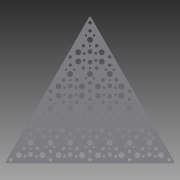
# Autodesk Inventor part: grid16-lightpipe
Saved by Autodesk Inventor 2013 (Build 170138000, 138)
## iProperties
Created: 2013-03-05
Part Number: grid16-lightpipe
Material: Generic
Document SubType Name: Modeling
Designer: Beth Scott
Density: 1 g/cm^3
Author: Beth Scott
Autodesk Inventor part; units mm, degrees
(part 1 of 2)
ref_plane "YZ Plane" through (0, 0, 0) normal (1, 0, 0) x (0, 1, 0)
ref_plane "XZ Plane" through (0, 0, 0) normal (0, 1, 0) x (-1, 0, 0)
ref_plane "XY Plane" through (0, 0, 0) normal (0, 0, 1) x (1, 0, 0)
sketch "Triangle 1mm" plane through (0, 0, 0) normal (0, 0, 1) x (1, 0, 0)
  line L0 (0, 0) -> (16.6665, 28.8672) construction
  line L1 (16.6665, 28.8672) -> (33.333, 0) construction
  line L2 (33.333, 0) -> (0, 0) construction
  line L3 (33.333, 0) -> (8.3332, 14.4336) construction
  line L4 (0, 0) -> (24.9997, 14.4336) construction
  line L5 (16.6665, 28.8672) -> (16.6665, 0) construction
  line L6 (0, 14.4336) -> (33.333, 14.4336) construction
  line L7 (0, 19.4336) -> (33.333, 19.4336) construction
  line L8 (0, 9.4336) -> (33.333, 9.4336) construction
  line L9 (16.6665, 19.4336) -> (16.6665, 14.4336) construction
  line L10 (16.6665, 14.4336) -> (16.6665, 9.4336) construction
  circle A0 centre (16.6665, 14.4336) radius 2.5
  circle A1 centre (16.6665, 14.4336) radius 14.4336 construction
  circle A2 centre (6.7821, 3.9156) radius 2.5
  circle A3 centre (26.5509, 3.9156) radius 2.5
  circle A4 centre (16.6665, 14.4336) radius 10 construction
  circle A5 centre (16.6665, 4.4336) radius 2
  circle A6 centre (16.6665, 14.4336) radius 7.5 construction
  circle A7 centre (11.0763, 9.4336) radius 1.5
  circle A8 centre (22.2567, 9.4336) radius 1.5
  circle A9 centre (16.6665, 9.4336) radius 1
  circle A10 centre (16.6665, 21.9336) radius 1.5
  circle A11 centre (16.6665, 14.4336) radius 5 construction
  line L11 (5.4465, 9.4336) -> (22.2567, 19.4336) construction
  line L12 (27.8865, 9.4336) -> (11.0763, 19.4336) construction
  circle A12 centre (20.046, 18.1186) radius 1
  circle A13 centre (13.287, 18.1186) radius 1
  circle A14 centre (16.6665, 14.4336) radius 12.5 construction
  circle A15 centre (21.5432, 2.9241) radius 1.25
  circle A16 centre (11.7898, 2.9241) radius 1.25
  line L13 (16.6665, 4.4336) -> (21.5432, 2.9241) construction
  line L14 (21.5432, 2.9241) -> (26.5509, 3.9156) construction
  line L15 (6.7821, 3.9156) -> (11.7898, 2.9241) construction
  line L16 (11.7898, 2.9241) -> (16.6665, 4.4336) construction
  circle A17 centre (0, 0) radius 2.75 construction
  circle A18 centre (33.333, 0) radius 2.75 construction
  circle A19 centre (16.6665, 28.8672) radius 2.75 construction
  point P0 (16.9666, 9.7956)
  dimension "d55" = 20
  dimension "d14" = 33.333
  dimension "d31" = 10
  dimension "d43" = 5
  dimension "d54" = 5
  dimension "d56" = 4
  dimension "d57" = 15
  dimension "d58" = 3
  dimension "d59" = 2
  dimension "d60" = 25
  dimension "d61" = 2.5
  dimension "d64" = 5.5
  measures "d14" distance of L1.end L0.start
  measures "d31" distance of L8.start L7.start
  measures "d43" diameter of A0
  measures "d54" diameter of A2
  measures "d56" diameter of A5
  measures "d57" diameter of A6
  measures "d58" diameter of A7
  measures "d59" diameter of A9
  measures "d60" diameter of A14
  measures "d61" diameter of A15
  measures "d64" diameter of A17
sketch "Tri16 1mm" plane through (0, 0, 0) normal (0, 0, 1) x (1, 0, 0)
  line L0 (0, 0) -> (16.6665, 28.8672) construction
  line L1 (16.6665, 28.8672) -> (33.333, 0) construction
  line L2 (33.333, 0) -> (0, 0) construction
  line L3 (33.333, 0) -> (8.3333, 14.4336) construction
  line L4 (0, 0) -> (24.9998, 14.4336) construction
  line L5 (16.6665, 28.8672) -> (16.6665, 0) construction
  line L6 (0, 14.4336) -> (33.333, 14.4336) construction
  line L7 (0, 19.4336) -> (33.333, 19.4336) construction
  line L8 (0, 9.4336) -> (33.333, 9.4336) construction
  line L9 (16.6665, 19.4336) -> (16.6665, 14.4336) construction
  line L10 (16.6665, 14.4336) -> (16.6665, 9.4336) construction
  circle A0 centre (16.6665, 14.4336) radius 2.5
  circle A1 centre (16.6665, 14.4336) radius 14.4336 construction
  circle A2 centre (6.7821, 3.9156) radius 2.5
  circle A3 centre (26.5509, 3.9156) radius 2.5
  circle A4 centre (16.6665, 14.4336) radius 10 construction
  circle A5 centre (16.6665, 4.4336) radius 2
  circle A6 centre (16.6665, 14.4336) radius 7.5 construction
  circle A7 centre (11.0763, 9.4336) radius 1.5
  circle A8 centre (22.2567, 9.4336) radius 1.5
  circle A9 centre (16.6665, 9.4336) radius 1
  circle A10 centre (16.6665, 21.9336) radius 1.5
  circle A11 centre (16.6665, 14.4336) radius 5 construction
  line L11 (5.4465, 9.4336) -> (22.2567, 19.4336) construction
  line L12 (27.8865, 9.4336) -> (11.0763, 19.4336) construction
  circle A12 centre (20.046, 18.1186) radius 1
  circle A13 centre (13.287, 18.1186) radius 1
  circle A14 centre (16.6665, 14.4336) radius 12.5 construction
  circle A15 centre (21.5432, 2.9241) radius 1.25
  circle A16 centre (11.7898, 2.9241) radius 1.25
  line L13 (16.6665, 4.4336) -> (21.5432, 2.9241) construction
  line L14 (21.5432, 2.9241) -> (26.5509, 3.9156) construction
  line L15 (6.7821, 3.9156) -> (11.7898, 2.9241) construction
  line L16 (11.7898, 2.9241) -> (16.6665, 4.4336) construction
  circle A17 centre (0, 0) radius 2.75 construction
  circle A18 centre (33.333, 0) radius 2.75 construction
  circle A19 centre (16.6665, 28.8672) radius 2.75 construction
  line L17 (33.333, 0) -> (49.9995, 28.8672) construction
  line L18 (49.9995, 28.8672) -> (66.666, 0) construction
  line L19 (66.666, 0) -> (33.333, 0) construction
  line L20 (66.666, 0) -> (41.6663, 14.4336) construction
  line L21 (33.333, 0) -> (58.3328, 14.4336) construction
  line L22 (49.9995, 28.8672) -> (49.9995, 0) construction
  line L23 (33.333, 14.4336) -> (66.666, 14.4336) construction
  line L24 (33.333, 19.4336) -> (66.666, 19.4336) construction
  line L25 (33.333, 9.4336) -> (66.666, 9.4336) construction
  line L26 (49.9995, 19.4336) -> (49.9995, 14.4336) construction
  line L27 (49.9995, 14.4336) -> (49.9995, 9.4336) construction
  circle A20 centre (49.9995, 14.4336) radius 2.5
  circle A21 centre (49.9995, 14.4336) radius 14.4336 construction
  circle A22 centre (40.1151, 3.9156) radius 2.5
  circle A23 centre (59.8839, 3.9156) radius 2.5
  circle A24 centre (49.9995, 14.4336) radius 10 construction
  circle A25 centre (49.9995, 4.4336) radius 2
  circle A26 centre (49.9995, 14.4336) radius 7.5 construction
  circle A27 centre (44.4093, 9.4336) radius 1.5
  circle A28 centre (55.5897, 9.4336) radius 1.5
  circle A29 centre (49.9995, 9.4336) radius 1
  circle A30 centre (49.9995, 21.9336) radius 1.5
  circle A31 centre (49.9995, 14.4336) radius 5 construction
  line L28 (38.7795, 9.4336) -> (55.5897, 19.4336) construction
  line L29 (61.2195, 9.4336) -> (44.4093, 19.4336) construction
  circle A32 centre (53.379, 18.1186) radius 1
  circle A33 centre (46.62, 18.1186) radius 1
  circle A34 centre (49.9995, 14.4336) radius 12.5 construction
  circle A35 centre (54.8762, 2.9241) radius 1.25
  circle A36 centre (45.1228, 2.9241) radius 1.25
  line L30 (49.9995, 4.4336) -> (54.8762, 2.9241) construction
  line L31 (54.8762, 2.9241) -> (59.8839, 3.9156) construction
  line L32 (40.1151, 3.9156) -> (45.1228, 2.9241) construction
  line L33 (45.1228, 2.9241) -> (49.9995, 4.4336) construction
  circle A37 centre (33.333, 0) radius 2.75 construction
  circle A38 centre (66.666, 0) radius 2.75 construction
  circle A39 centre (49.9995, 28.8672) radius 2.75 construction
  line L34 (49.9995, 28.8672) -> (33.333, 0) construction
  line L35 (33.333, 0) -> (16.6665, 28.8672) construction
  line L36 (16.6665, 28.8672) -> (49.9995, 28.8672) construction
  line L37 (16.6665, 28.8672) -> (41.6663, 14.4336) construction
  line L38 (49.9995, 28.8672) -> (24.9998, 14.4336) construction
  line L39 (33.333, 0) -> (33.333, 28.8672) construction
  line L40 (49.9995, 14.4336) -> (16.6665, 14.4336) construction
  line L41 (49.9995, 9.4336) -> (16.6665, 9.4336) construction
  line L42 (49.9995, 19.4336) -> (16.6665, 19.4336) construction
  line L43 (33.333, 9.4336) -> (33.333, 14.4336) construction
  line L44 (33.333, 14.4336) -> (33.333, 19.4336) construction
  circle A40 centre (33.333, 14.4336) radius 2.5
  circle A41 centre (33.333, 14.4336) radius 14.4336 construction
  circle A42 centre (43.2174, 24.9516) radius 2.5
  circle A43 centre (23.4486, 24.9516) radius 2.5
  circle A44 centre (33.333, 14.4336) radius 10 construction
  circle A45 centre (33.333, 24.4336) radius 2
  circle A46 centre (33.333, 14.4336) radius 7.5 construction
  circle A47 centre (38.9232, 19.4336) radius 1.5
  circle A48 centre (27.7428, 19.4336) radius 1.5
  circle A49 centre (33.333, 19.4336) radius 1
  circle A50 centre (33.333, 6.9336) radius 1.5
  circle A51 centre (33.333, 14.4336) radius 5 construction
  line L45 (44.553, 19.4336) -> (27.7428, 9.4336) construction
  line L46 (22.113, 19.4336) -> (38.9232, 9.4336) construction
  circle A52 centre (29.9535, 10.7487) radius 1
  circle A53 centre (36.7125, 10.7487) radius 1
  circle A54 centre (33.333, 14.4336) radius 12.5 construction
  circle A55 centre (28.4563, 25.9431) radius 1.25
  circle A56 centre (38.2097, 25.9431) radius 1.25
  line L47 (33.333, 24.4336) -> (28.4563, 25.9431) construction
  line L48 (28.4563, 25.9431) -> (23.4486, 24.9516) construction
  line L49 (43.2174, 24.9516) -> (38.2097, 25.9431) construction
  line L50 (38.2097, 25.9431) -> (33.333, 24.4336) construction
  circle A57 centre (49.9995, 28.8672) radius 2.75 construction
  circle A58 centre (16.6665, 28.8672) radius 2.75 construction
  circle A59 centre (33.333, 0) radius 2.75 construction
  line L51 (83.3325, 28.8672) -> (66.666, 0) construction
  line L52 (66.666, 0) -> (49.9995, 28.8672) construction
  line L53 (49.9995, 28.8672) -> (83.3325, 28.8672) construction
  line L54 (49.9995, 28.8672) -> (74.9993, 14.4336) construction
  line L55 (83.3325, 28.8672) -> (58.3328, 14.4336) construction
  line L56 (66.666, 0) -> (66.666, 28.8672) construction
  line L57 (83.3325, 14.4336) -> (49.9995, 14.4336) construction
  line L58 (83.3325, 9.4336) -> (49.9995, 9.4336) construction
  line L59 (83.3325, 19.4336) -> (49.9995, 19.4336) construction
  line L60 (66.666, 9.4336) -> (66.666, 14.4336) construction
  line L61 (66.666, 14.4336) -> (66.666, 19.4336) construction
  circle A60 centre (66.666, 14.4336) radius 2.5
  circle A61 centre (66.666, 14.4336) radius 14.4336 construction
  circle A62 centre (76.5504, 24.9516) radius 2.5
  circle A63 centre (56.7816, 24.9516) radius 2.5
  circle A64 centre (66.666, 14.4336) radius 10 construction
  circle A65 centre (66.666, 24.4336) radius 2
  circle A66 centre (66.666, 14.4336) radius 7.5 construction
  circle A67 centre (72.2562, 19.4336) radius 1.5
  circle A68 centre (61.0758, 19.4336) radius 1.5
  circle A69 centre (66.666, 19.4336) radius 1
  circle A70 centre (66.666, 6.9336) radius 1.5
  circle A71 centre (66.666, 14.4336) radius 5 construction
  line L62 (77.886, 19.4336) -> (61.0758, 9.4336) construction
  line L63 (55.446, 19.4336) -> (72.2562, 9.4336) construction
  circle A72 centre (63.2865, 10.7487) radius 1
  circle A73 centre (70.0455, 10.7487) radius 1
  circle A74 centre (66.666, 14.4336) radius 12.5 construction
  circle A75 centre (61.7893, 25.9431) radius 1.25
  circle A76 centre (71.5427, 25.9431) radius 1.25
  line L64 (66.666, 24.4336) -> (61.7893, 25.9431) construction
  line L65 (61.7893, 25.9431) -> (56.7816, 24.9516) construction
  line L66 (76.5504, 24.9516) -> (71.5427, 25.9431) construction
  line L67 (71.5427, 25.9431) -> (66.666, 24.4336) construction
  circle A77 centre (83.3325, 28.8672) radius 2.75 construction
  circle A78 centre (49.9995, 28.8672) radius 2.75 construction
  circle A79 centre (66.666, 0) radius 2.75 construction
  line L68 (66.666, 0) -> (83.3325, 28.8672) construction
  line L69 (83.3325, 28.8672) -> (99.999, 0) construction
  line L70 (99.999, 0) -> (66.666, 0) construction
  line L71 (99.999, 0) -> (74.9993, 14.4336) construction
  line L72 (66.666, 0) -> (91.6658, 14.4336) construction
  line L73 (83.3325, 28.8672) -> (83.3325, 0) construction
  line L74 (66.666, 14.4336) -> (99.999, 14.4336) construction
  line L75 (66.666, 19.4336) -> (99.999, 19.4336) construction
  line L76 (66.666, 9.4336) -> (99.999, 9.4336) construction
  line L77 (83.3325, 19.4336) -> (83.3325, 14.4336) construction
  line L78 (83.3325, 14.4336) -> (83.3325, 9.4336) construction
  circle A80 centre (83.3325, 14.4336) radius 2.5
  circle A81 centre (83.3325, 14.4336) radius 14.4336 construction
  circle A82 centre (73.4481, 3.9156) radius 2.5
  circle A83 centre (93.2169, 3.9156) radius 2.5
  circle A84 centre (83.3325, 14.4336) radius 10 construction
  circle A85 centre (83.3325, 4.4336) radius 2
  circle A86 centre (83.3325, 14.4336) radius 7.5 construction
  circle A87 centre (77.7423, 9.4336) radius 1.5
  circle A88 centre (88.9227, 9.4336) radius 1.5
  circle A89 centre (83.3325, 9.4336) radius 1
  circle A90 centre (83.3325, 21.9336) radius 1.5
  circle A91 centre (83.3325, 14.4336) radius 5 construction
  line L79 (72.1125, 9.4336) -> (88.9227, 19.4336) construction
  line L80 (94.5525, 9.4336) -> (77.7423, 19.4336) construction
  circle A92 centre (86.712, 18.1186) radius 1
  circle A93 centre (79.953, 18.1186) radius 1
  circle A94 centre (83.3325, 14.4336) radius 12.5 construction
  circle A95 centre (88.2092, 2.9241) radius 1.25
  circle A96 centre (78.4558, 2.9241) radius 1.25
  line L81 (83.3325, 4.4336) -> (88.2092, 2.9241) construction
  line L82 (88.2092, 2.9241) -> (93.2169, 3.9156) construction
  line L83 (73.4481, 3.9156) -> (78.4558, 2.9241) construction
  line L84 (78.4558, 2.9241) -> (83.3325, 4.4336) construction
  circle A97 centre (66.666, 0) radius 2.75 construction
  circle A98 centre (99.999, 0) radius 2.75 construction
  circle A99 centre (83.3325, 28.8672) radius 2.75 construction
  line L85 (99.999, 0) -> (116.6655, 28.8672) construction
  line L86 (116.6655, 28.8672) -> (133.332, 0) construction
  line L87 (133.332, 0) -> (99.999, 0) construction
  line L88 (133.332, 0) -> (108.3323, 14.4336) construction
  line L89 (99.999, 0) -> (124.9988, 14.4336) construction
  line L90 (116.6655, 28.8672) -> (116.6655, 0) construction
  line L91 (99.999, 14.4336) -> (133.332, 14.4336) construction
  line L92 (99.999, 19.4336) -> (133.332, 19.4336) construction
  line L93 (99.999, 9.4336) -> (133.332, 9.4336) construction
  line L94 (116.6655, 19.4336) -> (116.6655, 14.4336) construction
  line L95 (116.6655, 14.4336) -> (116.6655, 9.4336) construction
  circle A100 centre (116.6655, 14.4336) radius 2.5
  circle A101 centre (116.6655, 14.4336) radius 14.4336 construction
  circle A102 centre (106.7811, 3.9156) radius 2.5
  circle A103 centre (126.5499, 3.9156) radius 2.5
  circle A104 centre (116.6655, 14.4336) radius 10 construction
  circle A105 centre (116.6655, 4.4336) radius 2
  circle A106 centre (116.6655, 14.4336) radius 7.5 construction
  circle A107 centre (111.0753, 9.4336) radius 1.5
  circle A108 centre (122.2557, 9.4336) radius 1.5
  circle A109 centre (116.6655, 9.4336) radius 1
  circle A110 centre (116.6655, 21.9336) radius 1.5
  circle A111 centre (116.6655, 14.4336) radius 5 construction
  line L96 (105.4455, 9.4336) -> (122.2557, 19.4336) construction
  line L97 (127.8855, 9.4336) -> (111.0753, 19.4336) construction
  circle A112 centre (120.045, 18.1186) radius 1
  circle A113 centre (113.286, 18.1186) radius 1
  circle A114 centre (116.6655, 14.4336) radius 12.5 construction
  circle A115 centre (121.5422, 2.9241) radius 1.25
  circle A116 centre (111.7888, 2.9241) radius 1.25
  line L98 (116.6655, 4.4336) -> (121.5422, 2.9241) construction
  line L99 (121.5422, 2.9241) -> (126.5499, 3.9156) construction
  line L100 (106.7811, 3.9156) -> (111.7888, 2.9241) construction
  line L101 (111.7888, 2.9241) -> (116.6655, 4.4336) construction
  circle A117 centre (99.999, 0) radius 2.75 construction
  circle A118 centre (133.332, 0) radius 2.75 construction
  circle A119 centre (116.6655, 28.8672) radius 2.75 construction
  line L102 (116.6655, 28.8672) -> (99.999, 0) construction
  line L103 (99.999, 0) -> (83.3325, 28.8672) construction
  line L104 (83.3325, 28.8672) -> (116.6655, 28.8672) construction
  line L105 (83.3325, 28.8672) -> (108.3323, 14.4336) construction
  line L106 (116.6655, 28.8672) -> (91.6658, 14.4336) construction
  line L107 (99.999, 0) -> (99.999, 28.8672) construction
  line L108 (116.6655, 14.4336) -> (83.3325, 14.4336) construction
  line L109 (116.6655, 9.4336) -> (83.3325, 9.4336) construction
  line L110 (116.6655, 19.4336) -> (83.3325, 19.4336) construction
  line L111 (99.999, 9.4336) -> (99.999, 14.4336) construction
  line L112 (99.999, 14.4336) -> (99.999, 19.4336) construction
  circle A120 centre (99.999, 14.4336) radius 2.5
  circle A121 centre (99.999, 14.4336) radius 14.4336 construction
  circle A122 centre (109.8834, 24.9516) radius 2.5
  circle A123 centre (90.1146, 24.9516) radius 2.5
  circle A124 centre (99.999, 14.4336) radius 10 construction
  circle A125 centre (99.999, 24.4336) radius 2
  circle A126 centre (99.999, 14.4336) radius 7.5 construction
  circle A127 centre (105.5892, 19.4336) radius 1.5
  circle A128 centre (94.4088, 19.4336) radius 1.5
  circle A129 centre (99.999, 19.4336) radius 1
  circle A130 centre (99.999, 6.9336) radius 1.5
  circle A131 centre (99.999, 14.4336) radius 5 construction
  line L113 (111.219, 19.4336) -> (94.4088, 9.4336) construction
  line L114 (88.779, 19.4336) -> (105.5892, 9.4336) construction
  circle A132 centre (96.6195, 10.7487) radius 1
  circle A133 centre (103.3785, 10.7487) radius 1
  circle A134 centre (99.999, 14.4336) radius 12.5 construction
  circle A135 centre (95.1223, 25.9431) radius 1.25
  circle A136 centre (104.8757, 25.9431) radius 1.25
  line L115 (99.999, 24.4336) -> (95.1223, 25.9431) construction
  line L116 (95.1223, 25.9431) -> (90.1146, 24.9516) construction
  line L117 (109.8834, 24.9516) -> (104.8757, 25.9431) construction
  line L118 (104.8757, 25.9431) -> (99.999, 24.4336) construction
  circle A137 centre (116.6655, 28.8672) radius 2.75 construction
  circle A138 centre (83.3325, 28.8672) radius 2.75 construction
  circle A139 centre (99.999, 0) radius 2.75 construction
  line L119 (16.6665, 28.8672) -> (33.333, 57.7344) construction
  line L120 (33.333, 57.7344) -> (49.9995, 28.8672) construction
  line L121 (49.9995, 28.8672) -> (16.6665, 28.8672) construction
  line L122 (49.9995, 28.8672) -> (24.9998, 43.3008) construction
  line L123 (16.6665, 28.8672) -> (41.6663, 43.3008) construction
  line L124 (33.333, 57.7344) -> (33.333, 28.8672) construction
  line L125 (16.6665, 43.3008) -> (49.9995, 43.3008) construction
  line L126 (16.6665, 48.3008) -> (49.9995, 48.3008) construction
  line L127 (16.6665, 38.3008) -> (49.9995, 38.3008) construction
  line L128 (33.333, 48.3008) -> (33.333, 43.3008) construction
  line L129 (33.333, 43.3008) -> (33.333, 38.3008) construction
  circle A140 centre (33.333, 43.3008) radius 2.5
  circle A141 centre (33.333, 43.3008) radius 14.4336 construction
  circle A142 centre (23.4486, 32.7829) radius 2.5
  circle A143 centre (43.2174, 32.7829) radius 2.5
  circle A144 centre (33.333, 43.3008) radius 10 construction
  circle A145 centre (33.333, 33.3008) radius 2
  circle A146 centre (33.333, 43.3008) radius 7.5 construction
  circle A147 centre (27.7428, 38.3008) radius 1.5
  circle A148 centre (38.9232, 38.3008) radius 1.5
  circle A149 centre (33.333, 38.3008) radius 1
  circle A150 centre (33.333, 50.8008) radius 1.5
  circle A151 centre (33.333, 43.3008) radius 5 construction
  line L130 (22.113, 38.3008) -> (38.9232, 48.3008) construction
  line L131 (44.553, 38.3008) -> (27.7428, 48.3008) construction
  circle A152 centre (36.7125, 46.9858) radius 1
  circle A153 centre (29.9535, 46.9858) radius 1
  circle A154 centre (33.333, 43.3008) radius 12.5 construction
  circle A155 centre (38.2097, 31.7914) radius 1.25
  circle A156 centre (28.4563, 31.7914) radius 1.25
  line L132 (33.333, 33.3008) -> (38.2097, 31.7914) construction
  line L133 (38.2097, 31.7914) -> (43.2174, 32.7829) construction
  line L134 (23.4486, 32.7829) -> (28.4563, 31.7914) construction
  line L135 (28.4563, 31.7914) -> (33.333, 33.3008) construction
  circle A157 centre (16.6665, 28.8672) radius 2.75 construction
  circle A158 centre (49.9995, 28.8672) radius 2.75 construction
  circle A159 centre (33.333, 57.7344) radius 2.75 construction
  line L136 (33.333, 57.7344) -> (49.9995, 86.6017) construction
  line L137 (49.9995, 86.6017) -> (66.666, 57.7344) construction
  line L138 (66.666, 57.7344) -> (33.333, 57.7344) construction
  line L139 (66.666, 57.7344) -> (41.6663, 72.1681) construction
  line L140 (33.333, 57.7344) -> (58.3328, 72.1681) construction
  line L141 (49.9995, 86.6017) -> (49.9995, 57.7344) construction
  line L142 (33.333, 72.1681) -> (66.666, 72.1681) construction
  line L143 (33.333, 77.1681) -> (66.666, 77.1681) construction
  line L144 (33.333, 67.1681) -> (66.666, 67.1681) construction
  line L145 (49.9995, 77.1681) -> (49.9995, 72.1681) construction
  line L146 (49.9995, 72.1681) -> (49.9995, 67.1681) construction
  circle A160 centre (49.9995, 72.1681) radius 2.5
  circle A161 centre (49.9995, 72.1681) radius 14.4336 construction
  circle A162 centre (40.1151, 61.6501) radius 2.5
  circle A163 centre (59.8839, 61.6501) radius 2.5
  circle A164 centre (49.9995, 72.1681) radius 10 construction
  circle A165 centre (49.9995, 62.1681) radius 2
  circle A166 centre (49.9995, 72.1681) radius 7.5 construction
  circle A167 centre (44.4093, 67.1681) radius 1.5
  circle A168 centre (55.5897, 67.1681) radius 1.5
  circle A169 centre (49.9995, 67.1681) radius 1
  circle A170 centre (49.9995, 79.6681) radius 1.5
  circle A171 centre (49.9995, 72.1681) radius 5 construction
  line L147 (38.7795, 67.1681) -> (55.5897, 77.1681) construction
  line L148 (61.2195, 67.1681) -> (44.4093, 77.1681) construction
  circle A172 centre (53.379, 75.853) radius 1
  circle A173 centre (46.62, 75.853) radius 1
  circle A174 centre (49.9995, 72.1681) radius 12.5 construction
  circle A175 centre (54.8762, 60.6586) radius 1.25
  circle A176 centre (45.1228, 60.6586) radius 1.25
  line L149 (49.9995, 62.1681) -> (54.8762, 60.6586) construction
  line L150 (54.8762, 60.6586) -> (59.8839, 61.6501) construction
  line L151 (40.1151, 61.6501) -> (45.1228, 60.6586) construction
  line L152 (45.1228, 60.6586) -> (49.9995, 62.1681) construction
  circle A177 centre (33.333, 57.7344) radius 2.75 construction
  circle A178 centre (66.666, 57.7344) radius 2.75 construction
  circle A179 centre (49.9995, 86.6017) radius 2.75 construction
  line L153 (49.9995, 86.6017) -> (66.666, 115.4689) construction
  line L154 (66.666, 115.4689) -> (83.3325, 86.6017) construction
  line L155 (83.3325, 86.6017) -> (49.9995, 86.6017) construction
  line L156 (83.3325, 86.6017) -> (58.3328, 101.0353) construction
  line L157 (49.9995, 86.6017) -> (74.9993, 101.0353) construction
  line L158 (66.666, 115.4689) -> (66.666, 86.6017) construction
  line L159 (49.9995, 101.0353) -> (83.3325, 101.0353) construction
  line L160 (49.9995, 106.0353) -> (83.3325, 106.0353) construction
  line L161 (49.9995, 96.0353) -> (83.3325, 96.0353) construction
  line L162 (66.666, 106.0353) -> (66.666, 101.0353) construction
  line L163 (66.666, 101.0353) -> (66.666, 96.0353) construction
  circle A180 centre (66.666, 101.0353) radius 2.5
  circle A181 centre (66.666, 101.0353) radius 14.4336 construction
  circle A182 centre (56.7816, 90.5173) radius 2.5
  circle A183 centre (76.5504, 90.5173) radius 2.5
  circle A184 centre (66.666, 101.0353) radius 10 construction
  circle A185 centre (66.666, 91.0353) radius 2
  circle A186 centre (66.666, 101.0353) radius 7.5 construction
  circle A187 centre (61.0758, 96.0353) radius 1.5
  circle A188 centre (72.2562, 96.0353) radius 1.5
  circle A189 centre (66.666, 96.0353) radius 1
  circle A190 centre (66.666, 108.5353) radius 1.5
  circle A191 centre (66.666, 101.0353) radius 5 construction
  line L164 (55.446, 96.0353) -> (72.2562, 106.0353) construction
  line L165 (77.886, 96.0353) -> (61.0758, 106.0353) construction
  circle A192 centre (70.0455, 104.7202) radius 1
  circle A193 centre (63.2865, 104.7202) radius 1
  circle A194 centre (66.666, 101.0353) radius 12.5 construction
  circle A195 centre (71.5427, 89.5258) radius 1.25
  circle A196 centre (61.7893, 89.5258) radius 1.25
  line L166 (66.666, 91.0353) -> (71.5427, 89.5258) construction
  line L167 (71.5427, 89.5258) -> (76.5504, 90.5173) construction
  line L168 (56.7816, 90.5173) -> (61.7893, 89.5258) construction
  line L169 (61.7893, 89.5258) -> (66.666, 91.0353) construction
  circle A197 centre (49.9995, 86.6017) radius 2.75 construction
  circle A198 centre (83.3325, 86.6017) radius 2.75 construction
  circle A199 centre (66.666, 115.4689) radius 2.75 construction
  line L170 (66.666, 57.7344) -> (49.9995, 28.8672) construction
  line L171 (49.9995, 28.8672) -> (33.333, 57.7344) construction
  line L172 (33.333, 57.7344) -> (66.666, 57.7344) construction
  line L173 (33.333, 57.7344) -> (58.3328, 43.3008) construction
  line L174 (66.666, 57.7344) -> (41.6663, 43.3008) construction
  line L175 (49.9995, 28.8672) -> (49.9995, 57.7344) construction
  line L176 (66.666, 43.3008) -> (33.333, 43.3008) construction
  line L177 (66.666, 38.3008) -> (33.333, 38.3008) construction
  line L178 (66.666, 48.3008) -> (33.333, 48.3008) construction
  line L179 (49.9995, 38.3008) -> (49.9995, 43.3008) construction
  line L180 (49.9995, 43.3008) -> (49.9995, 48.3008) construction
  circle A200 centre (49.9995, 43.3008) radius 2.5
  circle A201 centre (49.9995, 43.3008) radius 14.4336 construction
  circle A202 centre (59.8839, 53.8188) radius 2.5
  circle A203 centre (40.1151, 53.8188) radius 2.5
  circle A204 centre (49.9995, 43.3008) radius 10 construction
  circle A205 centre (49.9995, 53.3008) radius 2
  circle A206 centre (49.9995, 43.3008) radius 7.5 construction
  circle A207 centre (55.5897, 48.3008) radius 1.5
  circle A208 centre (44.4093, 48.3008) radius 1.5
  circle A209 centre (49.9995, 48.3008) radius 1
  circle A210 centre (49.9995, 35.8008) radius 1.5
  circle A211 centre (49.9995, 43.3008) radius 5 construction
  line L181 (61.2195, 48.3008) -> (44.4093, 38.3008) construction
  line L182 (38.7795, 48.3008) -> (55.5897, 38.3008) construction
  circle A212 centre (46.62, 39.6159) radius 1
  circle A213 centre (53.379, 39.6159) radius 1
  circle A214 centre (49.9995, 43.3008) radius 12.5 construction
  circle A215 centre (45.1228, 54.8103) radius 1.25
  circle A216 centre (54.8762, 54.8103) radius 1.25
  line L183 (49.9995, 53.3008) -> (45.1228, 54.8103) construction
  line L184 (45.1228, 54.8103) -> (40.1151, 53.8188) construction
  line L185 (59.8839, 53.8188) -> (54.8762, 54.8103) construction
  line L186 (54.8762, 54.8103) -> (49.9995, 53.3008) construction
  circle A217 centre (66.666, 57.7344) radius 2.75 construction
  circle A218 centre (33.333, 57.7344) radius 2.75 construction
  circle A219 centre (49.9995, 28.8672) radius 2.75 construction
  line L187 (83.3325, 86.6017) -> (66.666, 57.7344) construction
  line L188 (66.666, 57.7344) -> (49.9995, 86.6017) construction
  line L189 (49.9995, 86.6017) -> (83.3325, 86.6017) construction
  line L190 (49.9995, 86.6017) -> (74.9993, 72.1681) construction
  line L191 (83.3325, 86.6017) -> (58.3328, 72.1681) construction
  line L192 (66.666, 57.7344) -> (66.666, 86.6017) construction
  line L193 (83.3325, 72.1681) -> (49.9995, 72.1681) construction
  line L194 (83.3325, 67.1681) -> (49.9995, 67.1681) construction
  line L195 (83.3325, 77.1681) -> (49.9995, 77.1681) construction
  line L196 (66.666, 67.1681) -> (66.666, 72.1681) construction
  line L197 (66.666, 72.1681) -> (66.666, 77.1681) construction
  circle A220 centre (66.666, 72.1681) radius 2.5
  circle A221 centre (66.666, 72.1681) radius 14.4336 construction
  circle A222 centre (76.5504, 82.686) radius 2.5
  circle A223 centre (56.7816, 82.686) radius 2.5
  circle A224 centre (66.666, 72.1681) radius 10 construction
  circle A225 centre (66.666, 82.1681) radius 2
  circle A226 centre (66.666, 72.1681) radius 7.5 construction
  circle A227 centre (72.2562, 77.1681) radius 1.5
  circle A228 centre (61.0758, 77.1681) radius 1.5
  circle A229 centre (66.666, 77.1681) radius 1
  circle A230 centre (66.666, 64.6681) radius 1.5
  circle A231 centre (66.666, 72.1681) radius 5 construction
  line L198 (77.886, 77.1681) -> (61.0758, 67.1681) construction
  line L199 (55.446, 77.1681) -> (72.2562, 67.1681) construction
  circle A232 centre (63.2865, 68.4831) radius 1
  circle A233 centre (70.0455, 68.4831) radius 1
  circle A234 centre (66.666, 72.1681) radius 12.5 construction
  circle A235 centre (61.7893, 83.6775) radius 1.25
  circle A236 centre (71.5427, 83.6775) radius 1.25
  line L200 (66.666, 82.1681) -> (61.7893, 83.6775) construction
  line L201 (61.7893, 83.6775) -> (56.7816, 82.686) construction
  line L202 (76.5504, 82.686) -> (71.5427, 83.6775) construction
  line L203 (71.5427, 83.6775) -> (66.666, 82.1681) construction
  circle A237 centre (83.3325, 86.6017) radius 2.75 construction
  circle A238 centre (49.9995, 86.6017) radius 2.75 construction
  circle A239 centre (66.666, 57.7344) radius 2.75 construction
  line L204 (66.666, 57.7344) -> (83.3325, 86.6017) construction
  line L205 (83.3325, 86.6017) -> (99.999, 57.7344) construction
  line L206 (99.999, 57.7344) -> (66.666, 57.7344) construction
  line L207 (99.999, 57.7344) -> (74.9993, 72.1681) construction
  line L208 (66.666, 57.7344) -> (91.6658, 72.1681) construction
  line L209 (83.3325, 86.6017) -> (83.3325, 57.7344) construction
  line L210 (66.666, 72.1681) -> (99.999, 72.1681) construction
  line L211 (66.666, 77.1681) -> (99.999, 77.1681) construction
  line L212 (66.666, 67.1681) -> (99.999, 67.1681) construction
  line L213 (83.3325, 77.1681) -> (83.3325, 72.1681) construction
  line L214 (83.3325, 72.1681) -> (83.3325, 67.1681) construction
  circle A240 centre (83.3325, 72.1681) radius 2.5
  circle A241 centre (83.3325, 72.1681) radius 14.4336 construction
  circle A242 centre (73.4481, 61.6501) radius 2.5
  circle A243 centre (93.2169, 61.6501) radius 2.5
  circle A244 centre (83.3325, 72.1681) radius 10 construction
  circle A245 centre (83.3325, 62.1681) radius 2
  circle A246 centre (83.3325, 72.1681) radius 7.5 construction
  circle A247 centre (77.7423, 67.1681) radius 1.5
  circle A248 centre (88.9227, 67.1681) radius 1.5
  circle A249 centre (83.3325, 67.1681) radius 1
  circle A250 centre (83.3325, 79.6681) radius 1.5
  circle A251 centre (83.3325, 72.1681) radius 5 construction
  line L215 (72.1125, 67.1681) -> (88.9227, 77.1681) construction
  line L216 (94.5525, 67.1681) -> (77.7423, 77.1681) construction
  circle A252 centre (86.712, 75.853) radius 1
  circle A253 centre (79.953, 75.853) radius 1
  circle A254 centre (83.3325, 72.1681) radius 12.5 construction
  circle A255 centre (88.2092, 60.6586) radius 1.25
  circle A256 centre (78.4558, 60.6586) radius 1.25
  line L217 (83.3325, 62.1681) -> (88.2092, 60.6586) construction
  line L218 (88.2092, 60.6586) -> (93.2169, 61.6501) construction
  line L219 (73.4481, 61.6501) -> (78.4558, 60.6586) construction
  line L220 (78.4558, 60.6586) -> (83.3325, 62.1681) construction
  circle A257 centre (66.666, 57.7344) radius 2.75 construction
  circle A258 centre (99.999, 57.7344) radius 2.75 construction
  circle A259 centre (83.3325, 86.6017) radius 2.75 construction
  line L221 (49.9995, 28.8672) -> (66.666, 57.7344) construction
  line L222 (66.666, 57.7344) -> (83.3325, 28.8672) construction
  line L223 (83.3325, 28.8672) -> (49.9995, 28.8672) construction
  line L224 (83.3325, 28.8672) -> (58.3328, 43.3008) construction
  line L225 (49.9995, 28.8672) -> (74.9993, 43.3008) construction
  line L226 (66.666, 57.7344) -> (66.666, 28.8672) construction
  line L227 (49.9995, 43.3008) -> (83.3325, 43.3008) construction
  line L228 (49.9995, 48.3008) -> (83.3325, 48.3008) construction
  line L229 (49.9995, 38.3008) -> (83.3325, 38.3008) construction
  line L230 (66.666, 48.3008) -> (66.666, 43.3008) construction
  line L231 (66.666, 43.3008) -> (66.666, 38.3008) construction
  circle A260 centre (66.666, 43.3008) radius 2.5
  circle A261 centre (66.666, 43.3008) radius 14.4336 construction
  circle A262 centre (56.7816, 32.7829) radius 2.5
  circle A263 centre (76.5504, 32.7829) radius 2.5
  circle A264 centre (66.666, 43.3008) radius 10 construction
  circle A265 centre (66.666, 33.3008) radius 2
  circle A266 centre (66.666, 43.3008) radius 7.5 construction
  circle A267 centre (61.0758, 38.3008) radius 1.5
  circle A268 centre (72.2562, 38.3008) radius 1.5
  circle A269 centre (66.666, 38.3008) radius 1
  circle A270 centre (66.666, 50.8008) radius 1.5
  circle A271 centre (66.666, 43.3008) radius 5 construction
  line L232 (55.446, 38.3008) -> (72.2562, 48.3008) construction
  line L233 (77.886, 38.3008) -> (61.0758, 48.3008) construction
  circle A272 centre (70.0455, 46.9858) radius 1
  circle A273 centre (63.2865, 46.9858) radius 1
  circle A274 centre (66.666, 43.3008) radius 12.5 construction
  circle A275 centre (71.5427, 31.7914) radius 1.25
  circle A276 centre (61.7893, 31.7914) radius 1.25
  line L234 (66.666, 33.3008) -> (71.5427, 31.7914) construction
  line L235 (71.5427, 31.7914) -> (76.5504, 32.7829) construction
  line L236 (56.7816, 32.7829) -> (61.7893, 31.7914) construction
  line L237 (61.7893, 31.7914) -> (66.666, 33.3008) construction
  circle A277 centre (49.9995, 28.8672) radius 2.75 construction
  circle A278 centre (83.3325, 28.8672) radius 2.75 construction
  circle A279 centre (66.666, 57.7344) radius 2.75 construction
  line L238 (83.3325, 28.8672) -> (99.999, 57.7344) construction
  line L239 (99.999, 57.7344) -> (116.6655, 28.8672) construction
  line L240 (116.6655, 28.8672) -> (83.3325, 28.8672) construction
  line L241 (116.6655, 28.8672) -> (91.6658, 43.3008) construction
  line L242 (83.3325, 28.8672) -> (108.3323, 43.3008) construction
  line L243 (99.999, 57.7344) -> (99.999, 28.8672) construction
  line L244 (83.3325, 43.3008) -> (116.6655, 43.3008) construction
  line L245 (83.3325, 48.3008) -> (116.6655, 48.3008) construction
  line L246 (83.3325, 38.3008) -> (116.6655, 38.3008) construction
  line L247 (99.999, 48.3008) -> (99.999, 43.3008) construction
  line L248 (99.999, 43.3008) -> (99.999, 38.3008) construction
  circle A280 centre (99.999, 43.3008) radius 2.5
  circle A281 centre (99.999, 43.3008) radius 14.4336 construction
  circle A282 centre (90.1146, 32.7829) radius 2.5
  circle A283 centre (109.8834, 32.7829) radius 2.5
  circle A284 centre (99.999, 43.3008) radius 10 construction
  circle A285 centre (99.999, 33.3008) radius 2
  circle A286 centre (99.999, 43.3008) radius 7.5 construction
  circle A287 centre (94.4088, 38.3008) radius 1.5
  circle A288 centre (105.5892, 38.3008) radius 1.5
  circle A289 centre (99.999, 38.3008) radius 1
  circle A290 centre (99.999, 50.8008) radius 1.5
  circle A291 centre (99.999, 43.3008) radius 5 construction
  line L249 (88.779, 38.3008) -> (105.5892, 48.3008) construction
  line L250 (111.219, 38.3008) -> (94.4088, 48.3008) construction
  circle A292 centre (103.3785, 46.9858) radius 1
  circle A293 centre (96.6195, 46.9858) radius 1
  circle A294 centre (99.999, 43.3008) radius 12.5 construction
  circle A295 centre (104.8757, 31.7914) radius 1.25
  circle A296 centre (95.1223, 31.7914) radius 1.25
  line L251 (99.999, 33.3008) -> (104.8757, 31.7914) construction
  line L252 (104.8757, 31.7914) -> (109.8834, 32.7829) construction
  line L253 (90.1146, 32.7829) -> (95.1223, 31.7914) construction
  line L254 (95.1223, 31.7914) -> (99.999, 33.3008) construction
  circle A297 centre (83.3325, 28.8672) radius 2.75 construction
  circle A298 centre (116.6655, 28.8672) radius 2.75 construction
  circle A299 centre (99.999, 57.7344) radius 2.75 construction
  line L255 (99.999, 57.7344) -> (83.3325, 28.8672) construction
  line L256 (83.3325, 28.8672) -> (66.666, 57.7344) construction
  line L257 (66.666, 57.7344) -> (99.999, 57.7344) construction
  line L258 (66.666, 57.7344) -> (91.6658, 43.3008) construction
  line L259 (99.999, 57.7344) -> (74.9993, 43.3008) construction
  line L260 (83.3325, 28.8672) -> (83.3325, 57.7344) construction
  line L261 (99.999, 43.3008) -> (66.666, 43.3008) construction
  line L262 (99.999, 38.3008) -> (66.666, 38.3008) construction
  line L263 (99.999, 48.3008) -> (66.666, 48.3008) construction
  line L264 (83.3325, 38.3008) -> (83.3325, 43.3008) construction
  line L265 (83.3325, 43.3008) -> (83.3325, 48.3008) construction
  circle A300 centre (83.3325, 43.3008) radius 2.5
  circle A301 centre (83.3325, 43.3008) radius 14.4336 construction
  circle A302 centre (93.2169, 53.8188) radius 2.5
  circle A303 centre (73.4481, 53.8188) radius 2.5
  circle A304 centre (83.3325, 43.3008) radius 10 construction
  circle A305 centre (83.3325, 53.3008) radius 2
  circle A306 centre (83.3325, 43.3008) radius 7.5 construction
  circle A307 centre (88.9227, 48.3008) radius 1.5
  circle A308 centre (77.7423, 48.3008) radius 1.5
  circle A309 centre (83.3325, 48.3008) radius 1
  circle A310 centre (83.3325, 35.8008) radius 1.5
  circle A311 centre (83.3325, 43.3008) radius 5 construction
  line L266 (94.5525, 48.3008) -> (77.7423, 38.3008) construction
  line L267 (72.1125, 48.3008) -> (88.9227, 38.3008) construction
  circle A312 centre (79.953, 39.6159) radius 1
  circle A313 centre (86.712, 39.6159) radius 1
  circle A314 centre (83.3325, 43.3008) radius 12.5 construction
  circle A315 centre (78.4558, 54.8103) radius 1.25
  circle A316 centre (88.2092, 54.8103) radius 1.25
  line L268 (83.3325, 53.3008) -> (78.4558, 54.8103) construction
  line L269 (78.4558, 54.8103) -> (73.4481, 53.8188) construction
  line L270 (93.2169, 53.8188) -> (88.2092, 54.8103) construction
  line L271 (88.2092, 54.8103) -> (83.3325, 53.3008) construction
  circle A317 centre (99.999, 57.7344) radius 2.75 construction
  circle A318 centre (66.666, 57.7344) radius 2.75 construction
  circle A319 centre (83.3325, 28.8672) radius 2.75 construction
  point P0 (66.741, 38.5329)